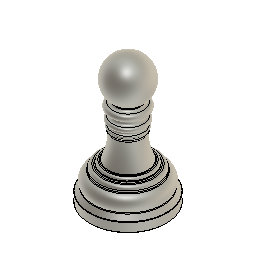
Pawn Target v6 (Autodesk Fusion 360 design; units mm, degrees)
Autodesk Fusion 360 part; units mm, degrees
sketch "Sketch2" plane through (0, 0, 0) normal (0, 1, 0) x (1, 0, 0)
  line L0 (0, 0) -> (45.72, 0)
  line L1 (45.72, 0) -> (45.72, -11.43)
  line L2 (45.72, -11.43) -> (40.3156, -16.8344)
  arc A0 (34.29, -33.02) -> (40.3156, -16.8344) centre (31.75, -22.86) ccw
  arc A1 (23.495, -43.815) -> (17.145, -73.66) centre (90.4558, -73.66) ccw
  line L3 (18.034, -72.39) -> (18.034, -124.46)
  circle A2 centre (18.034, -79.121) radius 1.27
  circle A3 centre (18.034, -76.835) radius 1.016
  circle A4 centre (18.034, -82.296) radius 1.905
  circle A5 centre (18.034, -86.741) radius 2.54
  circle A6 centre (18.034, -92.456) radius 3.175
  circle A7 centre (18.034, -99.441) radius 3.81
  circle A8 centre (18.034, -107.061) radius 3.81
  line L4 (0, 0) -> (0, -177.8)
  circle A9 centre (0, -127) radius 25.4
  line L5 (34.29, -33.02) -> (34.29, -35.56)
  arc A10 (30.48, -39.37) -> (34.29, -35.56) centre (30.48, -35.56) ccw
  line L6 (27.94, -39.37) -> (30.48, -39.37)
  line L7 (27.94, -41.275) -> (27.94, -39.37)
  arc A11 (25.4, -43.815) -> (27.94, -41.275) centre (25.4, -41.275) ccw
  line L8 (23.495, -43.815) -> (25.4, -43.815)
  circle A12 centre (18.034, -75.184) radius 0.635
  arc A13 (17.145, -73.66) -> (18.034, -74.549) centre (18.034, -73.66) ccw
  line L9 (17.145, -73.66) -> (17.145, -74.295) construction
  point P0 (18.034, -74.549)
  dimension "d5" = 135
  dimension "d6" = 45.72
  dimension "d7" = 11.43
  dimension "d10" = 34.29
  dimension "d11" = 33.02
  dimension "d12" = 31.75
  dimension "d13" = 22.86
  dimension "d18" = 2.54
  dimension "d19" = 2.032
  dimension "d20" = 3.81
  dimension "d21" = 5.08
  dimension "d22" = 6.35
  dimension "d23" = 7.62
  dimension "d24" = 2.286
  dimension "d25" = 3.175
  dimension "d26" = 4.445
  dimension "d27" = 5.715
  dimension "d28" = 6.985
  dimension "d29" = 7.62
  dimension "d30" = 7.62
  dimension "d31" = 50.8
  dimension "d32" = 127
  dimension "d35" = 2.54
  dimension "d36" = 1.905
  dimension "d37" = 2.54
  dimension "d38" = 1.905
  dimension "d39" = 3.81
  dimension "d40" = 2.54
  dimension "d42" = 1.27
  dimension "d43" = 1.651
  dimension "d44" = 17.145
  dimension "d45" = 73.66
  dimension "d51" = 0.889
  constraint coincident L0.start L4.start
  constraint horizontal L0
  constraint perpendicular L0 L1
  constraint vertical L3
  constraint coincident L3 A3.centre
  constraint coincident L3 A2.centre
  constraint coincident L3 A4.centre
  constraint coincident L3 A5.centre
  constraint coincident L3 A6.centre
  constraint coincident L3 A7.centre
  constraint coincident L3 A8.centre
  constraint perpendicular L0 L4
  constraint coincident L4 A9.centre
  constraint vertical L5
  constraint tangent L5 A10
  constraint tangent A10 L6
  constraint tangent L7 A11
  constraint tangent A11 L8
  constraint horizontal L8
  constraint horizontal L6
  constraint vertical L7
  constraint coincident A1.start L8.start
  constraint coincident L3 A12.centre
  constraint coincident L3 P0
  constraint coincident A12 P0
  constraint coincident P0 A13.end
  constraint tangent A12 A13
  constraint tangent A1 L9
  constraint vertical L9
  constraint coincident A1.end A13.start
  constraint tangent A1 A13
  measures "d5" angle of L1 L2
  measures "d6" distance of L0.start L0.end
  measures "d7" distance of L0.end L1.end
  measures "d10" horizontal distance of L0.start A0.start
  measures "d11" vertical distance of L0.start A0.start
  measures "d12" horizontal distance of L0.start A0.centre
  measures "d13" vertical distance of L0.start A0.centre
  measures "d18" diameter of A2
  measures "d19" diameter of A3
  measures "d20" diameter of A4
  measures "d21" diameter of A5
  measures "d22" diameter of A6
  measures "d23" diameter of A7
  measures "d24" distance of A2.centre A3.centre
  measures "d25" distance of A2.centre A4.centre
  measures "d26" distance of A4.centre A5.centre
  measures "d27" distance of A5.centre A6.centre
  measures "d28" distance of A6.centre A7.centre
  measures "d29" diameter of A8
  measures "d30" distance of A7.centre A8.centre
  measures "d31" diameter of A9
  measures "d32" distance of L0.start A9.centre
  measures "d35" distance of A10.start L6.start
  measures "d36" distance of L6.start L7.start
  measures "d37" distance of A0.start L5.end
  measures "d38" distance of A11.start A1.start
  measures "d39" radius of A10
  measures "d40" radius of A11
  measures "d42" diameter of A12
  measures "d43" distance of A3.centre A12.centre
  measures "d44" horizontal distance of L0.start A1.end
  measures "d45" vertical distance of L0.start A1.end
  measures "d51" radius of A13
revolve "Revolve2" add sketch "Sketch2" angle 360 about axis through (0, 0, 0) along (0, 0, 1) contours L0 L1 L2 A0 A1 A2 A3 A4 A5 A6 A7 A8 L4 A9 L5 A10 L6 L7 A11 L8 A12 A13 | A8 L4 A9 | L3 A8 A9 | L3 A7 | L3 A7 | L3 A8 A9 | L3 A5 | L3 A5 | L3 A2 | L3 A2 | L3 A12 | L3 A12 picked at (16.9665, -109.1352) picked at (18.1911, -109.8619)
fillet "Fillet1" radius 0.889 6 edges at (-37.5873, -14.5787, 16.8344) (-31.9695, -12.3998, 33.02) (-26.0492, -10.1035, 39.37) (-21.905, -8.4962, 43.815) (-13.3889, -5.1931, 106.0494) (-42.626, -16.5331, 11.43)
chamfer "Chamfer1" distance 0.889 angle 45 1 edges at (-42.626, -16.5331, 0)
hole "Hole1" at (0, 0, 0) direction (0, 0, 1) diameter 5.1054 depth 25.4 tip angle 118
thread "Thread2" "ANSI Unified Screw Threads 0.25 1/4-20 UNC 3B"
pattern_linear "R-Pattern1" count 3 spacing 25.4 along (1, 0, 0) both ways count 3 spacing 25.4 along (0, 1, 0) both ways of "Hole1"
equation "Fillet = 0.035 in"
equation "d49 = Fillet"
equation "d50 = Chamfer"
equation "d51 = Fillet"
equation "Chamfer = 0.035 in"
